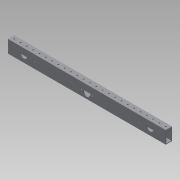
# Autodesk Inventor part: side rail
Saved by Autodesk Inventor 2015 (Build 190159000, 159)
## iProperties
Created: 2015-12-17
Part Number: side rail
Material: Generic
Document SubType Name: Modeling
Designer: Daniel
Density: 1 g/cm^3
Appearance: Default
Author: Daniel
Autodesk Inventor part; units mm, degrees
ref_plane "YZ Plane" through (0, 0, 0) normal (1, 0, 0) x (0, 1, 0)
ref_plane "XZ Plane" through (0, 0, 0) normal (0, 1, 0) x (-1, 0, 0)
ref_plane "XY Plane" through (0, 0, 0) normal (0, 0, 1) x (1, 0, 0)
sketch "Sketch1" plane through (0, 0, 0) normal (1, 0, 0) x (0, 1, 0)
  line L0 (0, 0) -> (50.8, 0)
  line L1 (50.8, 0) -> (50.8, 25.4)
  line L2 (50.8, 25.4) -> (0, 25.4)
  line L3 (0, 25.4) -> (0, 0)
  line L4 (2.54, 22.86) -> (48.26, 22.86)
  line L5 (48.26, 22.86) -> (48.26, 2.54)
  line L6 (48.26, 2.54) -> (2.54, 2.54)
  line L7 (2.54, 2.54) -> (2.54, 22.86)
  dimension "d0" = 50.8
  dimension "d1" = 25.4
  dimension "d2" = 2.54
  constraints: 16 end point, 4 parallel, 2 perpendicular, 1 horizontal, 3 other
  measures "d0" distance of L2.end L1.end
  measures "d1" distance of L1.end L0.end
  measures "d2" distance between parallel lines of L2 L4
extrude "Extrusion1" add sketch "Sketch1" along normal blind 635
sketch "Sketch2" plane through (0, 0, 25.4) normal (0, 0, 1) x (1, 0, 0)
  circle A0 centre (63.5254, 28.575) radius 14.2875
  line L0 (0, 50.8) -> (0, 0) projected
  line L1 (0, 50.8) -> (635, 50.8) projected
  line L2 (0, 0) -> (635, 0) projected
  circle A1 centre (571.4746, 28.575) radius 14.2875
  line L3 (635, 50.8) -> (635, 0) projected
  circle A2 centre (529.8186, 25.4) radius 1.5875
  circle A3 centre (105.1814, 25.4) radius 1.5875
  dimension "d5" = 28.575
  dimension "d6" = 63.5254
  dimension "d8" = 28.575
  dimension "d9" = 28.575
  dimension "d10" = 63.5254
  dimension "d11" = 28.575
  dimension "d12" = 3.175
  dimension "d13" = 41.656
  dimension "d14" = 3.175
  dimension "d15" = 41.656
  dimension "d16" = 25.4
  dimension "d17" = 25.4
  constraints: 4 centre point
  measures "d5" diameter of A0
  measures "d6" distance from line of L0 A0.centre
  measures "d8" distance from line of A0.centre L2
  measures "d9" diameter of A1
  measures "d10" distance from line of A1.centre L3
  measures "d11" distance from line of L2 A1.centre
  measures "d12" diameter of A2
  measures "d13" horizontal distance of A1.centre A2.centre
  measures "d14" diameter of A3
  measures "d15" horizontal distance of A0.centre A3.centre
  measures "d16" distance from line of L2 A3.centre
  measures "d17" distance from line of L2 A2.centre
extrude "Extrusion2" cut sketch "Sketch2" against normal through all contours A0 | A1 | A2 | A3
sketch "Sketch3" plane through (0, 0, 25.4) normal (0, 0, 1) x (1, 0, 0)
  circle A0 centre (317.5, 22.225) radius 14.2875
  line L0 (0, 50.8) -> (635, 50.8) projected
  circle A1 centre (294.9638, 22.225) radius 2.5527
  circle A2 centre (340.0361, 22.225) radius 2.5527
  point P0 (0, 0)
  point P1 (317.5, 50.8)
  dimension "d20" = 28.575
  dimension "d21" = 28.575
  dimension "d36" = 22.5361
  dimension "d37" = 22.5361
  dimension "d38" = 5.1054
  dimension "d39" = 5.1054
  constraints: 3 centre point, 2 coincident, 1 midpoint, 1 vertical alignment
  measures "d20" diameter of A0
  measures "d21" distance from line of L0 A0.centre
  measures "d36" distance of A0.centre point (294.964, 22.225)
  measures "d37" distance of A0.centre point (340.036, 22.225)
  measures "d38" diameter of A1
  measures "d39" diameter of A2
extrude "Extrusion3" cut sketch "Sketch3" against normal through all contours A0
sketch "Sketch4" plane through (0, 50.8, 25.4) normal (0, 1, 0) x (1, 0, 0)
  circle A0 centre (12.7, 12.7) radius 2.54
  line L0 (0, 25.4) -> (0, 0) projected
  line L1 (0, 25.4) -> (635, 25.4) projected
  circle A1 centre (38.1, 12.7) radius 2.54
  circle A2 centre (63.5, 12.7) radius 2.54
  circle A3 centre (88.9, 12.7) radius 2.54
  circle A4 centre (114.3, 12.7) radius 2.54
  circle A5 centre (139.7, 12.7) radius 2.54
  circle A6 centre (165.1, 12.7) radius 2.54
  circle A7 centre (190.5, 12.7) radius 2.54
  circle A8 centre (215.9, 12.7) radius 2.54
  circle A9 centre (241.3, 12.7) radius 2.54
  circle A10 centre (266.7, 12.7) radius 2.54
  circle A11 centre (292.1, 12.7) radius 2.54
  circle A12 centre (317.5, 12.7) radius 2.54
  circle A13 centre (342.9, 12.7) radius 2.54
  circle A14 centre (368.3, 12.7) radius 2.54
  circle A15 centre (393.7, 12.7) radius 2.54
  circle A16 centre (419.1, 12.7) radius 2.54
  circle A17 centre (444.5, 12.7) radius 2.54
  circle A18 centre (469.9, 12.7) radius 2.54
  circle A19 centre (495.3, 12.7) radius 2.54
  circle A20 centre (520.7, 12.7) radius 2.54
  circle A21 centre (546.1, 12.7) radius 2.54
  circle A22 centre (571.5, 12.7) radius 2.54
  circle A23 centre (596.9, 12.7) radius 2.54
  circle A24 centre (622.3, 12.7) radius 2.54
  dimension "d24" = 5.08
  dimension "d25" = 12.7
  dimension "d26" = 12.7
  dimension "d29" = 25.4
  constraints: 25 centre point, 1 horizontal, 48 other
  measures "d24" diameter of A0
  measures "d25" distance from line of L0 A0.centre
  measures "d26" distance from line of L1 A0.centre
  measures "d29" distance of A0.centre A1.centre
extrude "Extrusion4" cut sketch "Sketch4" against normal through all
sketch "Sketch5" plane through (0, 0, 25.4) normal (0, 0, 1) x (1, 0, 0)
  circle A0 centre (294.9638, 22.225) radius 2.54
  circle A1 centre (340.0361, 22.225) radius 2.54
  line L0 (0, 50.8) -> (635, 50.8) projected
  line L1 (294.9638, 22.225) -> (340.0361, 22.225) construction
  point P0 (0, 0)
  point P1 (317.5, 22.225)
  point P2 (317.5, 50.8)
  dimension "d40" = 5.08
  dimension "d41" = 5.08
  dimension "d42" = 28.575
  dimension "d43" = 28.575
  dimension "d44" = 45.0723
  constraints: 2 centre point, 2 end point, 2 midpoint, 1 vertical alignment
  measures "d40" diameter of A0
  measures "d41" diameter of A1
  measures "d42" distance from line of L0 L1.start
  measures "d43" distance from line of L0 L1.end
  measures "d44" distance of L1.start L1.end
extrude "Extrusion5" cut sketch "Sketch5" against normal through all
body "Solid1"
